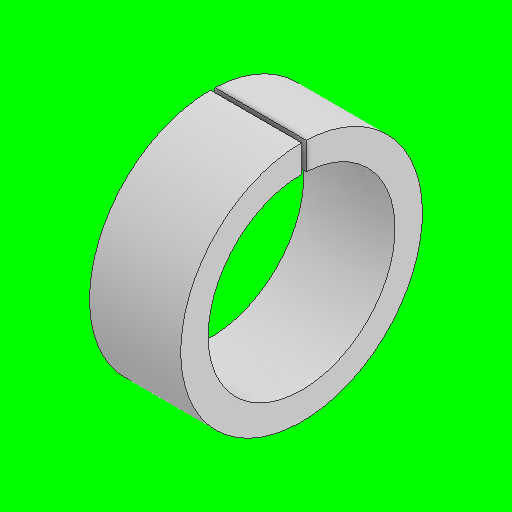
# Autodesk Inventor part: Spacer
Saved by Autodesk Inventor 2023 (Build 270158000, 158)
## iProperties
Created: 2022-03-29
Part Number: Spacer
Material: 一般
Document SubType Name: Modeling
Designer: neko2
Density: 1 g/cm^3
Appearance: 既定
Author: neko2
Autodesk Inventor part; units mm, degrees
ref_plane "YZ Plane" through (0, 0, 0) normal (1, 0, 0) x (0, 1, 0)
ref_plane "XZ Plane" through (0, 0, 0) normal (0, 1, 0) x (-1, 0, 0)
ref_plane "XY Plane" through (0, 0, 0) normal (0, 0, 1) x (1, 0, 0)
sketch "スケッチ1" plane through (0, 0, 0) normal (1, 0, 0) x (0, 1, 0)
  circle A0 centre (0, 0) radius 2.05
  arc A1 (2.65, 0) -> (2.6481, -0.1) centre (0, 0) ccw
  line L0 (2.65, 0) -> (2.05, 0)
  line L1 (2.6481, -0.1) -> (2.0476, -0.1)
  dimension "d1" = 4.1
  dimension "d4" = 2.65
  dimension "d5" = 0.1
  constraints: 4 end point, 4 point on circle, 2 centre point, 2 coincident, 1 horizontal, 1 horizontal alignment, 1 parallel
  measures "d1" diameter of A0
  measures "d4" radius of A1
  measures "d5" distance between parallel lines of L1 L0
extrude "押し出し1" add sketch "スケッチ1" along normal blind 2 contours A0 L1 A1 L0
